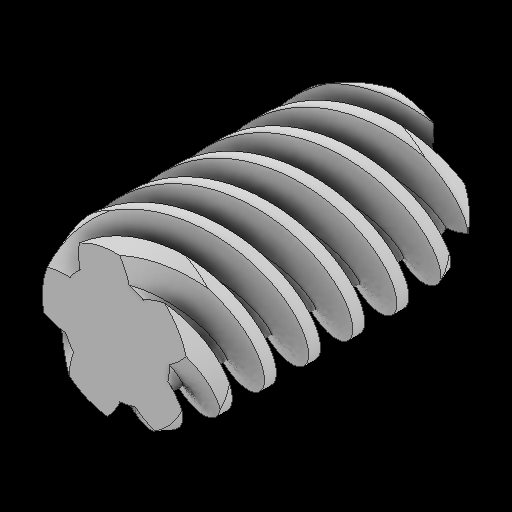
# Autodesk Inventor part: Tornillo_sin'
Saved by Autodesk Inventor 2027 (Build 310192000, 192)
## iProperties
Created: 2026-05-13
Part Number: Tornillo_sin'
Material: Genérico
Document SubType Name: Modeling
Designer: giova
Density: 1 g/cm^3
Appearance: Valor por defecto
Author: giova
Autodesk Inventor part; units mm, degrees
ref_plane "YZ Plane" through (0, 0, 0) normal (1, 0, 0) x (0, 1, 0)
ref_plane "XZ Plane" through (0, 0, 0) normal (0, 1, 0) x (-1, 0, 0)
ref_plane "XY Plane" through (0, 0, 0) normal (0, 0, 1) x (1, 0, 0)
sketch "Boceto1" plane through (0, 0, 0) normal (0, 0, 1) x (1, 0, 0)
  circle A0 centre (0, 0) radius 30
  dimension "d0" = 60
  constraints: 1 centre point, 1 coincident
  measures "d0" diameter of A0
extrude "Extrusión1" add sketch "Boceto1" along normal blind 100
sketch "Boceto2" plane through (0, 0, 100) normal (0, 0, 1) x (1, 0, 0)
  circle A0 centre (0, 0) radius 25
  dimension "d3" = 50
  constraints: 1 centre point, 1 coincident
  measures "d3" diameter of A0
surface extrude "SuperficieExtrusión1" sketch "Boceto2" against normal blind 100 shown no curves A0
chamfer "Chaflán1" distance 11 distance2 4 1 edges at (-30, 0, 100) measured on face at (29.9027, -2.414, 66.6667)
chamfer "Chaflán2" distance 11 distance2 4 1 edges at (-30, 0, 0) measured on face at (29.9027, -2.414, 59.3333)
sketch "Boceto3" plane through (0, 0, 0) normal (1, 0, 0) x (0, 1, 0)
  line L0 (30, 89) -> (-30, 89) projected
  line L1 (-30, 11) -> (30, 11) projected
  line L2 (0, 89) -> (0, 11) construction
  line L3 (30, 110.6979) -> (30, 99.2581)
  line L4 (30, 99.2581) -> (19.165, 103.2018)
  line L5 (19.165, 103.2018) -> (19.165, 106.7542)
  line L6 (19.165, 106.7542) -> (30, 110.6979)
  line L7 (25, 104.978) -> (25, 101.078) construction
  point P0 (0, 0)
  point P1 (30, 104.978)
  point P2 (0, 50)
  point P3 (30, 104.978)
  point P4 (19.165, 104.978)
  dimension "d12" = 54.978
  dimension "d13" = 110
  dimension "d14" = 30
  dimension "d15" = 19.165
  dimension "d16" = 25
  dimension "d17" = 3.9
  constraints: 12 end point, 5 midpoint, 2 horizontal alignment, 2 vertical, 1 coincident, 1 parallel, 1 point on line
  measures "d12" vertical distance of point (0, 50) point (30, 104.978)
  measures "d13" angle of L5 L6
  measures "d14" horizontal distance of point (0, 50) L3.start
  measures "d15" distance from line of point (0, 50) L5
  measures "d16" horizontal distance of point (0, 50) L7.start
  measures "d17" distance of L7.start L7.end
coil "Bobina1" sketch "Boceto3" operation cut axis through (0, 0, -10) along (0, 0, -1) pitch 78.5 turns 8 hand right
pattern_circular "Patrón circular1" count 5 over 360 about axis through (0, 0, -10) along (0, 0, 1) of "Bobina1"
